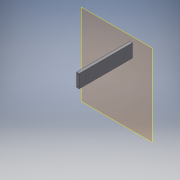
# Autodesk Inventor part: Z Stage_Linear Block Holder
Saved by Autodesk Inventor 2019 (Build 230136000, 136)
## iProperties
Created: 2020-03-07
Part Number: Z Stage_Linear Block Holder
Material: Generic
Document SubType Name: Modeling
Designer: Vijay
Density: 1 g/cm^3
Appearance: Default
Author: Vijay
Autodesk Inventor part; units mm, degrees
ref_plane "YZ Plane" through (0, 0, 0) normal (1, 0, 0) x (0, 1, 0)
ref_plane "XZ Plane" through (0, 0, 0) normal (0, 1, 0) x (-1, 0, 0)
ref_plane "Work Plane1" through (0, 0, 0) normal (0, 0, 1) x (1, 0, 0)
sketch "Sketch1" plane through (0, 0, 0) normal (0, 0, 1) x (1, 0, 0)
  line L0 (21.7578, -254.9236) -> (1.9524, -272.1401) projected
  line L1 (21.7578, -209.6761) -> (21.7578, -194.8761) projected
  line L2 (41.7578, 173.6589) -> (21.7578, 153.6589) projected
  line L3 (41.7578, 173.6589) -> (101.7578, 173.6589) projected
  line L4 (101.7578, 173.6589) -> (101.7578, 273.6589) projected
  line L5 (101.7578, 273.6589) -> (-10.4252, 273.6589) projected
  line L6 (-30.4252, 253.6589) -> (-10.4252, 273.6589) projected
  line L7 (-30.4252, 253.6589) -> (-30.4252, -206.3411) projected
  line L8 (-46.4251, -222.341) -> (-30.4252, -206.3411) projected
  line L9 (-260.4252, -226.3411) -> (-260.4252, -235.2654) projected
  line L10 (-260.4252, -235.2654) -> (1.9524, -272.1401) projected
  line L11 (101.7578, 173.6589) -> (81.7578, 173.6589)
  line L12 (81.7578, 173.6589) -> (81.7578, 273.6589)
  line L13 (81.7578, 273.6589) -> (101.7578, 273.6589)
  line L14 (101.7578, 273.6589) -> (101.7578, 173.6589)
  circle A0 centre (19.7578, -202.2762) radius 1.6 projected
  circle A1 centre (19.7578, 98.8927) radius 1.6 projected
  line L15 (21.7578, 91.4928) -> (21.7578, 106.2928) projected
  line L16 (21.7578, -188.4761) -> (21.7578, 85.0928) projected
  line L17 (21.7578, 112.6928) -> (21.7578, 153.6589) projected
  line L18 (-72.7251, -226.3411) -> (-78.6251, -226.3411) projected
  line L19 (-46.4251, -222.341) -> (-46.4251, -226.3411) projected
  line L20 (-78.6251, -219.9911) -> (-78.6251, -226.3411) projected
  line L21 (-84.6251, -219.9911) -> (-78.6251, -219.9911) projected
  line L22 (-84.6251, -226.3411) -> (-84.6251, -219.9911) projected
  line L23 (-84.6251, -226.3411) -> (-178.3768, -226.3411) projected
  line L24 (-178.3768, -219.9911) -> (-178.3768, -226.3411) projected
  line L25 (-184.3768, -219.9911) -> (-178.3768, -219.9911) projected
  line L26 (-184.3768, -226.3411) -> (-184.3768, -219.9911) projected
  line L27 (-184.3768, -226.3411) -> (-190.2768, -226.3411) projected
  line L28 (-193.6768, -226.3411) -> (-199.5768, -226.3411) projected
  line L29 (-199.5768, -219.9911) -> (-199.5768, -226.3411) projected
  line L30 (-205.5768, -219.9911) -> (-199.5768, -219.9911) projected
  line L31 (-205.5768, -226.3411) -> (-205.5768, -219.9911) projected
  line L32 (-205.5768, -226.3411) -> (-260.4252, -226.3411) projected
  line L33 (21.7578, -254.9236) -> (21.7578, -216.0761) projected
  line L34 (-46.4251, -226.3411) -> (-57.4251, -226.3411) projected
  line L35 (-57.4251, -219.9911) -> (-57.4251, -226.3411) projected
  line L36 (-63.4251, -219.9911) -> (-57.4251, -219.9911) projected
  line L37 (-63.4251, -226.3411) -> (-63.4251, -219.9911) projected
  line L38 (-63.4251, -226.3411) -> (-69.3251, -226.3411) projected
  line L39 (21.7578, -216.0761) -> (17.5578, -216.0761) projected
  line L40 (17.5578, -216.0761) -> (17.5578, -209.6761) projected
  line L41 (17.5578, -209.6761) -> (21.7578, -209.6761) projected
  line L42 (21.7578, -194.8761) -> (17.5578, -194.8761) projected
  line L43 (17.5578, -194.8761) -> (17.5578, -188.4761) projected
  line L44 (17.5578, -188.4761) -> (21.7578, -188.4761) projected
  line L45 (21.7578, 85.0928) -> (17.5578, 85.0928) projected
  line L46 (17.5578, 85.0928) -> (17.5578, 91.4928) projected
  line L47 (17.5578, 91.4928) -> (21.7578, 91.4928) projected
  line L48 (21.7578, 106.2928) -> (17.5578, 106.2928) projected
  line L49 (17.5578, 106.2928) -> (17.5578, 112.6928) projected
  line L50 (17.5578, 112.6928) -> (21.7578, 112.6928) projected
  circle A2 centre (91.7578, 263.6589) radius 3 projected
  circle A3 centre (91.7578, 183.6589) radius 3 projected
  line L51 (-69.3251, -226.3411) -> (-69.3251, -232.1411) projected
  line L52 (-69.3251, -232.1411) -> (-68.0751, -232.1411) projected
  line L53 (-68.0751, -232.1411) -> (-68.0751, -234.5411) projected
  line L54 (-68.0751, -234.5411) -> (-69.3251, -234.5411) projected
  line L55 (-69.3251, -234.5411) -> (-69.3251, -237.1911) projected
  line L56 (-69.3251, -237.1911) -> (-72.7251, -237.1911) projected
  line L57 (-72.7251, -237.1911) -> (-72.7251, -234.5411) projected
  line L58 (-72.7251, -234.5411) -> (-73.9751, -234.5411) projected
  line L59 (-73.9751, -234.5411) -> (-73.9751, -232.1411) projected
  line L60 (-73.9751, -232.1411) -> (-72.7251, -232.1411) projected
  line L61 (-72.7251, -232.1411) -> (-72.7251, -226.3411) projected
  line L62 (-190.2768, -226.3411) -> (-190.2768, -232.1411) projected
  line L63 (-190.2768, -232.1411) -> (-189.0268, -232.1411) projected
  line L64 (-189.0268, -232.1411) -> (-189.0268, -234.5411) projected
  line L65 (-189.0268, -234.5411) -> (-190.2768, -234.5411) projected
  line L66 (-190.2768, -234.5411) -> (-190.2768, -237.1911) projected
  line L67 (-190.2768, -237.1911) -> (-193.6768, -237.1911) projected
  line L68 (-193.6768, -237.1911) -> (-193.6768, -234.5411) projected
  line L69 (-193.6768, -234.5411) -> (-194.9268, -234.5411) projected
  line L70 (-194.9268, -234.5411) -> (-194.9268, -232.1411) projected
  line L71 (-194.9268, -232.1411) -> (-193.6768, -232.1411) projected
  line L72 (-193.6768, -232.1411) -> (-193.6768, -226.3411) projected
  point P0 (0, 0)
  point P1 (-50.4252, -226.3411)
  dimension "d0" = 20
  constraints: 8 end point, 2 parallel, 1 horizontal, 1 perpendicular, 1 point on line
  measures "d0" distance between parallel lines of L4 L12
ref_plane "Work Plane2" through (-260.4252, -272.1401, 400) normal (0, 0, -1) x (0, 1, 0)
extrude "Extrusion1" add sketch "Sketch1" along normal up to surface (400 mm away) contours L12 L5 L4 L3 | A2 | A3
sketch "Sketch2" plane through (81.7578, 173.6589, 0) normal (-1, 0, 0) x (0, 0, 1)
  circle A0 centre (49.5, 60) radius 1.75 construction
  circle A1 centre (69.5, 60) radius 1.75 construction
  circle A2 centre (49.5, 40) radius 1.5 construction
  circle A3 centre (69.5, 40) radius 1.75 construction
  circle A4 centre (350.5, 60) radius 1.5 construction
  circle A5 centre (330.5, 60) radius 1.75 construction
  circle A6 centre (330.5, 40) radius 1.5 construction
  circle A7 centre (350.5, 40) radius 1.75 construction
  circle A8 centre (49.5, 60) radius 1.5
  circle A9 centre (49.5, 40) radius 1.5
  circle A10 centre (69.5, 60) radius 1.5
  circle A11 centre (69.5, 40) radius 1.5
  circle A12 centre (330.5, 60) radius 1.5
  circle A13 centre (350.5, 60) radius 1.5
  circle A14 centre (330.5, 40) radius 1.5
  circle A15 centre (350.5, 40) radius 1.5
  point P0 (0, -173.6589)
  dimension "d3" = 3
  dimension "d4" = 3
  dimension "d5" = 3
  dimension "d6" = 3
  dimension "d7" = 3
  dimension "d8" = 3
  dimension "d9" = 3
  dimension "d10" = 3
  constraints: 8 centre point, 8 coincident
  measures "d3" diameter of A8
  measures "d4" diameter of A9
  measures "d5" diameter of A10
  measures "d6" diameter of A11
  measures "d7" diameter of A12
  measures "d8" diameter of A13
  measures "d9" diameter of A14
  measures "d10" diameter of A15
extrude "Extrusion2" cut sketch "Sketch2" against normal through all
sketch "Sketch3" plane through (81.7578, 173.6589, 0) normal (-1, 0, 0) x (0, 0, 1)
  circle A0 centre (330.5, 40) radius 1.5 projected
  circle A1 centre (330.5, 60) radius 1.5 projected
  circle A2 centre (69.5, 60) radius 1.5 projected
  circle A3 centre (49.5, 60) radius 1.5 projected
  circle A4 centre (49.5, 40) radius 1.5 projected
  circle A5 centre (69.5, 40) radius 1.5 projected
  circle A6 centre (350.5, 60) radius 1.5 projected
  circle A7 centre (350.5, 40) radius 1.5 projected
  line L0 (400, 100) -> (400, 0) projected
  line L1 (0, 100) -> (400, 100) projected
  line L2 (0, 100) -> (0, 0) projected
  line L3 (0, 0) -> (400, 0) projected
  circle A8 centre (49.5, 60) radius 1.5 projected
  circle A9 centre (49.5, 60) radius 4
  circle A10 centre (69.5, 60) radius 4
  circle A11 centre (49.5, 40) radius 4
  circle A12 centre (69.5, 40) radius 1.5 projected
  circle A13 centre (69.5, 40) radius 4
  circle A14 centre (330.5, 60) radius 4
  circle A15 centre (350.5, 60) radius 4
  circle A16 centre (330.5, 40) radius 4
  circle A17 centre (350.5, 40) radius 1.5 projected
  circle A18 centre (350.5, 40) radius 4
  point P0 (0, -173.6589)
  dimension "d13" = 8
  dimension "d14" = 8
  dimension "d15" = 8
  dimension "d16" = 8
  dimension "d17" = 8
  dimension "d18" = 8
  dimension "d19" = 8
  dimension "d20" = 8
  constraints: 8 centre point, 8 coincident
  measures "d13" diameter of A9
  measures "d14" diameter of A10
  measures "d15" diameter of A11
  measures "d16" diameter of A13
  measures "d17" diameter of A14
  measures "d18" diameter of A15
  measures "d19" diameter of A16
  measures "d20" diameter of A18
extrude "Extrusion3" cut sketch "Sketch3" against normal blind 5 contours A9 | A10 | A11 | A13 | A14 | A15 | A16 | A18
sketch "Sketch4" plane through (81.7578, 173.6589, 0) normal (-1, 0, 0) x (0, 0, 1)
  circle A0 centre (220, 90) radius 1.65 construction
  circle A1 centre (180, 90) radius 1.65 construction
  circle A2 centre (180, 90) radius 2
  circle A3 centre (220, 90) radius 2
  point P0 (0, -173.6589)
  dimension "d23" = 4
  dimension "d24" = 4
  constraints: 2 centre point, 2 coincident
  measures "d23" diameter of A2
  measures "d24" diameter of A3
extrude "Extrusion4" cut sketch "Sketch4" against normal through all
sketch "Sketch5" plane through (81.7578, 173.6589, 0) normal (-1, 0, 0) x (0, 0, 1)
  circle A0 centre (180, 90) radius 2 construction
  circle A1 centre (220, 90) radius 2 construction
  circle A2 centre (180, 90) radius 5
  circle A3 centre (220, 90) radius 5
  point P0 (0, -173.6589)
  dimension "d27" = 10
  dimension "d28" = 10
  constraints: 2 centre point, 2 coincident
  measures "d27" diameter of A2
  measures "d28" diameter of A3
extrude "Extrusion5" cut sketch "Sketch5" against normal blind 6
sketch "Sketch6" plane through (0, 0, 0) normal (0, 0, -1) x (-1, 0, 0)
  circle A0 centre (-91.7578, 263.6589) radius 3 construction
  circle A1 centre (-91.7578, 183.6589) radius 3 construction
  circle A2 centre (-91.7578, 263.6589) radius 2.5
  circle A3 centre (-91.7578, 183.6589) radius 2.5
  point P0 (0, 0)
  dimension "d31" = 5
  dimension "d32" = 5
  constraints: 2 centre point, 2 coincident
  measures "d31" diameter of A2
  measures "d32" diameter of A3
extrude "Extrusion6" cut sketch "Sketch6" against normal blind 20
thread "Thread1" size "12-24 UNC" class "2B" standard "ANSI Unified Screw Threads" full length
thread "Thread2" size "12-24 UNC" class "2B" standard "ANSI Unified Screw Threads" full length
sketch "Sketch7" plane through (81.7578, 173.6589, 400) normal (0, 0, 1) x (1, 0, 0)
  circle A0 centre (10, 90) radius 3 construction
  circle A1 centre (10, 10) radius 2.5 construction
  circle A2 centre (10, 90) radius 2.5
  circle A3 centre (10, 10) radius 2.5
  point P0 (-81.7578, -173.6589)
  dimension "d39" = 5
  dimension "d40" = 5
  constraints: 2 centre point, 2 coincident
  measures "d39" diameter of A2
  measures "d40" diameter of A3
extrude "Extrusion7" cut sketch "Sketch7" against normal blind 20
thread "Thread3" size "12-24 UNC" class "2B" standard "ANSI Unified Screw Threads" full length
thread "Thread4" size "12-24 UNC" class "2B" standard "ANSI Unified Screw Threads" full length
body "Solid1"
